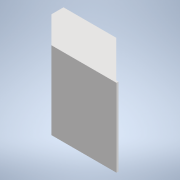
# Autodesk Inventor part: LPS_cap
Saved by Autodesk Inventor 2022 (Build 260153000, 153)
## iProperties
Created: 2024-07-06
Part Number: LPS_cap
Material: Типовые
Document SubType Name: Modeling
Designer: Капустяник Андрей
Density: 1 g/cm^3
Appearance: По умолчанию
Author: Капустяник Андрей
Autodesk Inventor part; units mm, degrees
ref_plane "YZ Plane" through (0, 0, 0) normal (1, 0, 0) x (0, 1, 0)
ref_plane "XZ Plane" through (0, 0, 0) normal (0, 1, 0) x (-1, 0, 0)
ref_plane "XY Plane" through (0, 0, 0) normal (0, 0, 1) x (1, 0, 0)
sketch "Эскиз1" plane through (0, 0, 0) normal (0, 0, 1) x (1, 0, 0)
  line L0 (-68.51, -58) -> (-68.51, 58) projected
  line L1 (-68.51, 58) -> (68.51, 58) projected
  line L2 (68.51, 58) -> (68.51, -58) projected
  line L3 (68.51, -58) -> (-68.51, -58) projected
  point P0 (0, 0)
extrude "Выдавливание1" add sketch "Эскиз1" along normal blind 3
sketch "Эскиз2" plane through (0, 0, 0) normal (0, 0, -1) x (-1, 0, 0)
  line L0 (-65.51, 55) -> (65.51, 55) projected
  line L1 (65.51, 55) -> (65.51, -55) projected
  line L2 (65.51, -55) -> (-65.51, -55) projected
  line L3 (-65.51, -55) -> (-65.51, 55) projected
  line L4 (68.51, -58) -> (68.51, 58) projected
  line L5 (68.51, 58) -> (-68.51, 58) projected
  line L6 (-68.51, 58) -> (-68.51, -58) projected
  line L7 (-68.51, -58) -> (68.51, -58) projected
  point P0 (0, 0)
ref_plane "РабПлоскость1" through (-68.51, -58, -55) normal (0, 0, 1) x (1, 0, 0)
extrude "Выдавливание2" add sketch "Эскиз2" along normal up to surface (55 mm away)
sketch "Эскиз3" plane through (-68.51, 58, 3) normal (0, 1, 0) x (1, 0, 0)
  line L0 (79.02, 58) -> (134.02, 3) projected
  line L1 (3, 3) -> (134.02, 3) projected
  line L2 (0, 58) -> (79.02, 58) projected
  line L3 (79.02, 58) -> (134.02, 3) projected
  line L4 (137.02, 3) -> (134.02, 3) projected
  line L5 (137.02, 3) -> (137.02, 76) projected
  line L6 (0, 76) -> (137.02, 76) projected
  line L7 (0, 58) -> (0, 76) projected
  line L8 (0, 58) -> (137.02, 58) projected
  line L9 (78.5957, 58) -> (133.8079, 2.7879)
  point P0 (68.51, 3)
  point P1 (133.5957, 3)
  dimension "d4" = 0.3
  constraints: 2 end point, 1 parallel, 1 point on line
  measures "d4" distance between parallel lines of L0 L9
extrude "Выдавливание3" cut sketch "Эскиз3" against normal up to surface (116 mm away) contours L8 L5 L4 L0 | L0 L1 L9 L2
chamfer "Фаска1" distance 40 angle 45 1 edges at (-68.51, 0, 3)
sketch "Эскиз4" plane through (-28.51, -58, 3) normal (-0.7071068, 0, 0.7071068) x (0.7071068, 0, 0.7071068)
  line L0 (-52.3259, 113) -> (-4.2426, 113) projected
  line L1 (-4.2426, 113) -> (-4.2426, 3) projected
  line L2 (-4.2426, 3) -> (-52.3259, 3) projected
  line L3 (-52.3259, 3) -> (-52.3259, 113) projected
  line L4 (-56.5685, 0) -> (0, 0) projected
  line L5 (0, 0) -> (0, 116) projected
  line L6 (0, 116) -> (-56.5685, 116) projected
  line L7 (-56.5685, 116) -> (-56.5685, 0) projected
  point P0 (18.0383, 58)
extrude "Выдавливание4" add sketch "Эскиз4" against normal blind 3 contours L0 L1 L2 L3 | L7 L6 L5 L4
sketch "Эскиз5" plane through (-28.51, -58, 3) normal (-0.7071068, 0, 0.7071068) x (0.7071068, 0, 0.7071068)
  line L0 (0, 116) -> (-56.5685, 116) projected
  line L1 (-56.5685, 116) -> (0, 116)
  line L2 (0, 116) -> (-28.2843, 116)
  line L3 (-56.5685, 116) -> (-28.2843, 116)
  line L4 (-42.4264, 116) -> (-42.4264, 0)
  line L5 (-56.5685, 0) -> (0, 0) projected
  line L6 (-42.4264, 58) -> (-42.4264, 116)
  line L7 (-42.4264, 87) -> (-42.4264, 116)
  line L8 (-42.4264, 58) -> (-42.4264, 0)
  line L9 (-42.4264, 29) -> (-42.4264, 0)
  circle A0 centre (-42.4264, 14.5) radius 2.5
  circle A1 centre (-42.4264, 29) radius 2.5
  circle A2 centre (-42.4264, 46) radius 5
  point P0 (18.0383, 58)
  dimension "d22" = 5
  dimension "d23" = 5
  dimension "d24" = 10
  constraints: 16 end point, 6 midpoint, 4 collinear, 3 centre point, 2 perpendicular, 2 point on line, 1 coincident, 1 horizontal
  measures "d22" diameter of A0
  measures "d23" diameter of A1
  measures "d24" diameter of A2
extrude "Выдавливание5" add sketch "Эскиз5" along normal blind 3
sketch "Эскиз7" plane through (-28.51, -58, 3) normal (-0.7071068, 0, 0.7071068) x (0.7071068, 0, 0.7071068)
  line L0 (-18.4, 103.5) -> (-37.6, 103.5)
  line L1 (-37.6, 103.5) -> (-37.6, 90.5)
  line L2 (-37.6, 90.5) -> (-18.4, 90.5)
  line L3 (-18.4, 90.5) -> (-18.4, 103.5)
  line L4 (-18.4, 103.5) -> (-37.6, 90.5) construction
  line L5 (-37.6, 103.5) -> (-18.4, 90.5) construction
  point P0 (18.0383, 58)
  point P1 (-28, 97)
  dimension "d20" = 19.2
  dimension "d21" = 13
  constraints: 12 end point, 2 midpoint, 2 parallel, 1 horizontal, 1 perpendicular
  measures "d20" distance of L2.end L1.end
  measures "d21" distance of L1.end L0.end
extrude "Выдавливание7" cut sketch "Эскиз7" against normal blind 3
sketch "Эскиз8" plane through (0, 0, 3) normal (0, 0, 1) x (1, 0, 0)
  line L0 (68.51, -58) -> (68.51, 58) projected
  line L1 (-28.51, -58) -> (-28.51, 58) projected
  line L2 (68.51, -58) -> (-28.51, 58)
  line L3 (-68.51, -58) -> (-28.51, -58) projected
  line L4 (68.51, 58) -> (-28.51, 58) projected
  line L5 (-28.51, -58) -> (68.51, 58)
  line L6 (-5, -25) -> (45, -25)
  line L7 (45, -25) -> (45, 25)
  line L8 (45, 25) -> (-5, 25)
  line L9 (-5, 25) -> (-5, -25)
  line L10 (-5, -25) -> (45, 25) construction
  line L11 (45, -25) -> (-5, 25) construction
  circle A0 centre (20, 0) radius 25
  point P0 (0, 0)
  dimension "d27" = 50
  dimension "d28" = 50
  constraints: 16 end point, 3 midpoint, 2 parallel, 1 centre point, 1 coincident, 1 horizontal, 1 perpendicular
  measures "d27" distance of L8.end L7.end
  measures "d28" distance of L7.end L6.end
extrude "Выдавливание8" cut sketch "Эскиз8" against normal blind 3 contours A0 L5 L2 | L2 L5 A0 | L5 L2 A0 | L5 A0 L2
